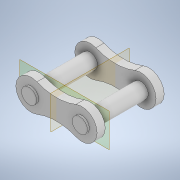
# Autodesk Inventor part: chain ink_outer
Saved by Autodesk Inventor 2022 (Build 260153000, 153)
## iProperties
Created: 2021-12-29
Part Number: chain ink_outer
Material: Generic
Document SubType Name: Modeling
Designer: MatusBarany
Density: 1 g/cm^3
Appearance: Default
Author: MatusBarany
Autodesk Inventor part; units mm, degrees
ref_plane "XZ Plane" through (0, 0, 0) normal (0, 1, 0) x (-1, 0, 0)
ref_plane "XY Plane" through (0, 0, 0) normal (0, 0, 1) x (1, 0, 0)
sketch "Sketch2" plane through (0, 0, 0) normal (0, 0, 1) x (1, 0, 0)
  circle A0 centre (2.5, 0) radius 1.5
  circle A1 centre (-2.5, 0) radius 1.5
  arc A2 (-1.9231, 1.3846) -> (1.9231, 1.3846) centre (0, 6) ccw
  arc A3 (1.9231, -1.3846) -> (-1.9231, -1.3846) centre (0, -6) ccw
  circle A4 centre (2.5, 0) radius 0.75
  circle A5 centre (-2.5, 0) radius 0.75
  point P0 (0, 0)
  dimension "d0" = 3
  dimension "d1" = 3
  dimension "d2" = 6
  dimension "d3" = 6
  dimension "d4" = 2.5
  dimension "d5" = 2.5
  dimension "d6" = 1.5
  dimension "d7" = 1.5
  constraints: 8 point on circle, 6 centre point, 4 tangent, 2 coincident, 2 horizontal alignment
  measures "d0" diameter of A1
  measures "d1" diameter of A0
  measures "d2" distance of A2.centre point (0, 0)
  measures "d3" distance of point (0, 0) A3.centre
  measures "d4" distance of point (0, 0) A0.centre
  measures "d5" distance of A1.centre point (0, 0)
  measures "d6" diameter of A5
  measures "d7" diameter of A4
extrude "Extrusion2" add sketch "Sketch2" along normal blind 0.8
ref_plane "Work Plane7" through (0, 0, 0) normal (0, 0, -1) x (-1, 0, 0)
sketch "Sketch9" plane through (0, 0, 0) normal (0, 0, -1) x (-1, 0, 0)
  arc A0 (1.9231, -1.3846) -> (-1.9231, -1.3846) centre (0, -6) ccw projected
  arc A1 (1.9231, -1.3846) -> (1.9231, 1.3846) centre (2.5, 0) ccw projected
  arc A2 (-1.9231, 1.3846) -> (1.9231, 1.3846) centre (0, 6) ccw projected
  arc A3 (-1.9231, 1.3846) -> (-1.9231, -1.3846) centre (-2.5, 0) ccw projected
  circle A4 centre (-2.5, 0) radius 0.75 projected
  circle A5 centre (2.5, 0) radius 0.75 projected
  circle A6 centre (-2.5, 0) radius 0.75
  point P0 (0, 0)
  constraints: 1 centre point, 1 coincident, 1 concentric
extrude "Extrusion8" add sketch "Sketch9" along normal blind 2.5 and the other way blind 1 contours A4
mirror "Mirror7" about plane through (0, 0, 0) normal (1, 0, 0) of "Extrusion8"
mirror "Mirror8" about plane through (-2.5, 0, -2.5) normal (0, 0, -1) of "Extrusion2", "Extrusion8", "Mirror7"
equation "\"d1\" = d0"
equation "\"d2\" = 2 * d0"
equation "\"d3\" = d2"
equation "\"d4\" = d5"
equation "\"d7\" = d6"
body "Solid2"
